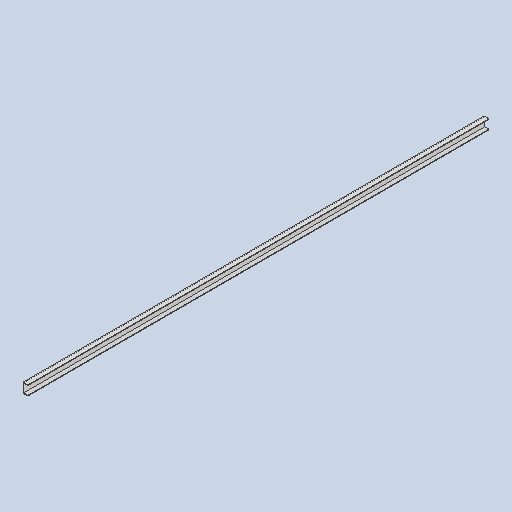
# Autodesk Inventor part: LongC96
Saved by Autodesk Inventor 2023 (Build 270158030, 158C)
## iProperties
Created: 2022-06-29
Part Number: LongC96
Material: Generic
Document SubType Name: Modeling
Designer: jeremyy
Density: 1 g/cm^3
Appearance: Default
Author: jeremyy
Autodesk Inventor part; units mm, degrees
ref_plane "YZ Plane" through (0, 0, 0) normal (1, 0, 0) x (0, 1, 0)
ref_plane "XZ Plane" through (0, 0, 0) normal (0, 1, 0) x (-1, 0, 0)
ref_plane "XY Plane" through (0, 0, 0) normal (0, 0, 1) x (1, 0, 0)
sketch "Sketch1" plane through (0, 0, 0) normal (0, 0, 1) x (1, 0, 0)
  line L0 (0, 0) -> (25.4, 0)
  line L1 (25.4, 0) -> (25.4, 3.175)
  line L2 (25.4, 3.175) -> (3.175, 3.175)
  line L3 (3.175, 3.175) -> (3.175, 47.625)
  line L4 (3.175, 47.625) -> (25.4, 47.625)
  line L5 (25.4, 47.625) -> (25.4, 50.8)
  line L6 (25.4, 50.8) -> (0, 50.8)
  line L7 (0, 50.8) -> (0, 0)
  dimension "d0" = 25.4
  dimension "d1" = 3.175
  dimension "d2" = 22.225
  dimension "d3" = 44.45
  dimension "d4" = 22.225
  dimension "d5" = 3.175
  constraints: 16 end point, 5 perpendicular, 2 point on line, 1 horizontal
  measures "d0" distance of L0.start L0.end
  measures "d1" distance of L0.end L1.end
  measures "d2" distance of L1.end L2.end
  measures "d3" distance of L2.end L3.end
  measures "d4" distance of L3.end L4.end
  measures "d5" distance of L4.end L5.end
extrude "Extrusion1" add sketch "Sketch1" along normal blind 2438.4
body "Solid1"
